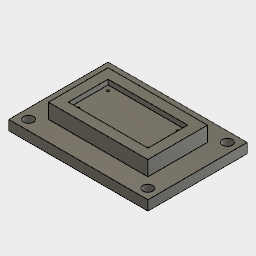
5V Power Converter v1 (Autodesk Fusion 360 design; units mm, degrees)
Autodesk Fusion 360 part; units mm, degrees
sketch "Sketch1" plane through (0, 0, 0) normal (0, 1, 0) x (1, 0, 0)
  line L0 (-48.26, 27.1965) -> (22.86, 27.1965)
  line L1 (22.86, 27.1965) -> (22.86, -23.6035)
  line L2 (22.86, -23.6035) -> (-48.26, -23.6035)
  line L3 (-48.26, -23.6035) -> (-48.26, 27.1965)
  dimension "d1" = 50.8
  dimension "d2" = 71.12
  constraint horizontal L0
  constraint vertical L1
  constraint horizontal L2
  constraint vertical L3
  measures "d17" distance of L1
  measures "d18" distance of L1
  measures "d19" distance of L1
  measures "d20" distance of L1
form "Form1" [no effect]
extrude "Extrude1" add sketch "Sketch1" along normal blind 5.08
sketch "Sketch2" plane through (0, 5.08, 0) normal (0, 1, 0) x (-1, 0, 0)
  line L0 (48.26, 23.6035) -> (-22.86, 23.6035)
  line L1 (-22.86, 23.6035) -> (-22.86, -27.1965)
  line L2 (-22.86, -27.1965) -> (48.26, -27.1965)
  line L3 (48.26, -27.1965) -> (48.26, 23.6035)
  line L4 (38.1, -17.0365) -> (-12.7, -17.0365)
  line L5 (-12.7, -17.0365) -> (-12.7, 13.4435)
  line L6 (-12.7, 13.4435) -> (38.1, 13.4435)
  line L7 (38.1, 13.4435) -> (38.1, -17.0365)
  dimension "d5" = 50.8
  dimension "d6" = 30.48
  dimension "d7" = 10.16
  dimension "d8" = 10.16
  constraint horizontal L4
  constraint vertical L5
  constraint horizontal L6
  constraint vertical L7
  measures "d6" distance of origin
  measures "d7" distance of L2 L4
  measures "d8" distance of L3 L7
extrude "Extrude2" add sketch "Sketch2" along normal blind 7.62 contours L4 L5 L6 L7
sketch "Sketch3" plane through (0, 12.7, 0) normal (0, 1, 0) x (-1, 0, 0)
  line L0 (38.1, 13.4435) -> (-12.7, 13.4435)
  line L1 (-12.7, 13.4435) -> (-12.7, -17.0365)
  line L2 (-12.7, -17.0365) -> (38.1, -17.0365)
  line L3 (38.1, -17.0365) -> (38.1, 13.4435)
  line L4 (33.02, -11.9565) -> (-7.62, -11.9565)
  line L5 (-7.62, -11.9565) -> (-7.62, 8.3635)
  line L6 (-7.62, 8.3635) -> (33.02, 8.3635)
  line L7 (33.02, 8.3635) -> (33.02, -11.9565)
  dimension "d11" = 40.64
  dimension "d12" = 20.32
  dimension "d13" = 5.08
  dimension "d14" = 5.08
  constraint horizontal L4
  constraint vertical L5
  constraint horizontal L6
  constraint vertical L7
  measures "d12" distance of origin
  measures "d13" distance of L2 L4
  measures "d14" distance of L3 L7
extrude "Extrude3" cut sketch "Sketch3" against normal blind 2.54 contours L4 L5 L6 L7
sketch "Sketch4" plane through (0, 5.08, 0) normal (0, 1, 0) x (-1, 0, 0)
  line L0 (38.1, 13.4435) -> (38.1, -17.0365)
  line L1 (38.1, -17.0365) -> (-12.7, -17.0365)
  line L2 (-12.7, -17.0365) -> (-12.7, 13.4435)
  line L3 (-12.7, 13.4435) -> (38.1, 13.4435)
  line L4 (48.26, 23.6035) -> (-22.86, 23.6035)
  line L5 (-22.86, 23.6035) -> (-22.86, -27.1965)
  line L6 (-22.86, -27.1965) -> (48.26, -27.1965)
  line L7 (48.26, -27.1965) -> (48.26, 23.6035)
  dimension "d17" = 5.08
  dimension "d18" = 5.08
  dimension "d19" = 5.08
  dimension "d20" = 5.08
  dimension "d21" = 5.08
  dimension "d22" = 5.08
  dimension "d23" = 5.08
  dimension "d24" = 5.08
  measures "d17" distance of L7 origin
  measures "d18" distance of L5 origin
  measures "d19" distance of L6 origin
  measures "d20" distance of L6 origin
  measures "d21" distance of L7
  measures "d22" distance of L4
  measures "d23" distance of L4
  measures "d24" distance of L5
hole "Hole1" at (17.78, 5.08, -22.1165) at (17.78, 5.08, 18.5235) at (-43.18, 5.08, 18.5235) at (-43.18, 5.08, -22.1165) direction (0, -1, 0) diameter 5.08 depth 40.64 tip angle 118
sketch "Sketch5" plane through (0, 10.16, 0) normal (0, 1, 0) x (-1, 0, 0)
  line L0 (33.02, 8.3635) -> (-7.62, 8.3635)
  line L1 (-7.62, 8.3635) -> (-7.62, -11.9565)
  line L2 (-7.62, -11.9565) -> (33.02, -11.9565)
  line L3 (33.02, -11.9565) -> (33.02, 8.3635)
  line L4 (-7.62, 8.3635) -> (33.02, 8.3635)
  line L5 (33.02, 8.3635) -> (33.02, -11.9565)
  line L6 (33.02, -11.9565) -> (-7.62, -11.9565)
  line L7 (-7.62, -11.9565) -> (-7.62, 8.3635)
  dimension "d28" = 2.54
  dimension "d29" = 2.54
  dimension "d30" = 2.54
  dimension "d31" = 2.54
  dimension "d32" = 2.54
  dimension "d33" = 2.54
  dimension "d34" = 2.54
  dimension "d35" = 2.54
  measures "d28" distance of origin L4
  measures "d29" distance of origin L5
  measures "d31" distance of L5
  measures "d33" distance of L7
  measures "d34" distance of origin L4
  measures "d35" distance of origin L7
hole "Hole2" at (-30.48, 10.16, -9.4165) at (5.08, 10.16, -9.4165) at (5.08, 10.16, 5.8235) at (-30.48, 10.16, 5.8235) direction (0, -1, 0) diameter 1.27 depth 50.8 tip angle 118
